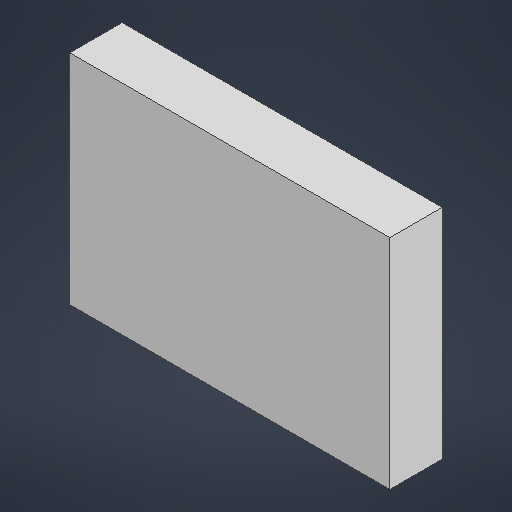
# Autodesk Inventor part: 斜板固定件
Saved by Autodesk Inventor 2025 (Build 290162000, 162)
## iProperties
Created: 2025-01-08
Part Number: 斜板固定件
Material: 常规
Document SubType Name: Modeling
Designer: HZD
Density: 1 g/cm^3
Appearance: 默认
Author: HZD
Autodesk Inventor part; units mm, degrees
ref_plane "YZ Plane" through (0, 0, 0) normal (1, 0, 0) x (0, 1, 0)
ref_plane "XZ Plane" through (0, 0, 0) normal (0, 1, 0) x (-1, 0, 0)
ref_plane "XY Plane" through (0, 0, 0) normal (0, 0, 1) x (1, 0, 0)
sketch "草图2" plane through (0, 0, 0) normal (0, 0, 1) x (1, 0, 0)
  line L0 (9.174, -6.2504) -> (-9.174, -6.2504)
  line L1 (-9.174, -6.2504) -> (-9.174, 6.2504)
  line L2 (-9.174, 6.2504) -> (9.174, 6.2504)
  line L3 (9.174, 6.2504) -> (9.174, -6.2504)
  line L4 (9.174, -6.2504) -> (-9.174, 6.2504) construction
  line L5 (-9.174, -6.2504) -> (9.174, 6.2504) construction
  point P0 (0, 0)
  constraints: 12 end point, 2 midpoint, 2 parallel, 1 horizontal, 1 perpendicular
extrude "拉伸1" add sketch "草图2" along normal blind 3
